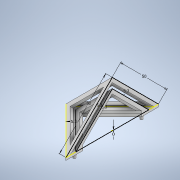
# Autodesk Inventor part: coltar5mmV3
Saved by Autodesk Inventor 2020 (Build 240168000, 168)
## iProperties
Created: 2022-02-13
Part Number: coltar5mmV3
Material: Generic
Document SubType Name: Modeling
Designer: Vlasciar
Density: 1 g/cm^3
Appearance: Default
Author: Vlasciar
Autodesk Inventor part; units mm, degrees
ref_plane "YZ Plane" through (0, 0, 0) normal (1, 0, 0) x (0, 1, 0)
ref_plane "XZ Plane" through (0, 0, 0) normal (0, 1, 0) x (-1, 0, 0)
ref_plane "XY Plane" through (0, 0, 0) normal (0, 0, 1) x (1, 0, 0)
sketch "Sketch2" plane through (0, 0, 0) normal (0, 1, 0) x (-1, 0, 0)
  line L0 (0, 35.355) -> (35.3557, 0)
  line L1 (35.3557, 0) -> (0, -35.355)
  line L2 (0, -35.355) -> (0, 35.355)
  point P0 (0, 0)
  point P1 (0, 0)
  dimension "d1" = 50
  dimension "d41" = 70.71
  constraints: 6 end point, 1 coincident, 1 equal length, 1 horizontal alignment, 1 midpoint
  measures "d1" distance of L0.start L0.end
  measures "d41" distance of L1.end L0.start
extrude "Extrusion1" add sketch "Sketch2" against normal blind 2
sketch "Sketch3" plane through (0, 0, 0) normal (0, 1, 0) x (1, 0, 0)
  line L0 (-35.3557, 0) -> (0, -35.355) projected
  line L1 (0, -35.355) -> (0, 35.355) projected
  line L2 (0, 35.355) -> (-35.3557, 0) projected
  point P0 (0, 0)
sketch "Sketch12" plane through (0, 0, 35.355) normal (1, 0, 0) x (0, 0, -1)
  line L0 (0, 0) -> (70.71, 0) projected
  line L1 (0, 0) -> (35.355, 35.3557)
  line L2 (35.355, 35.3557) -> (70.71, 0)
  line L3 (7.4953, 0) -> (63.2147, 0)
  line L4 (63.2147, 0) -> (35.355, 27.8603)
  line L5 (35.355, 27.8603) -> (7.4953, 0)
  point P0 (35.355, 0)
  dimension "d42" = 50
  dimension "d43" = 50
  dimension "d46" = 0
  dimension "d47" = 5.3
  dimension "d48" = 5.3
  constraints: 10 end point, 2 parallel, 1 horizontal
  measures "d42" distance of L1.end L0.end
  measures "d43" distance of L0.start L1.end
  measures "d46" distance between parallel lines of L0 L3
  measures "d47" distance between parallel lines of L2 L4
  measures "d48" distance between parallel lines of L1 L5
ref_plane "Work Plane5" through (-35.3557, 0, 0) normal (-0.5773466, 0.5773466, 0.5773577) x (0.7071136, 0, 0.7071)
ref_plane "Work Plane6" through (0, 0, -35.355) normal (0.5773466, -0.5773466, 0.5773577) x (-0.7071136, 0, 0.7071)
extrude "Extrusion10" add sketch "Sketch12" along normal up to surface surface through (-35.3557, 0, 0) normal (-0.5773466, 0.5773466, 0.5773577)
split "Split3" plane through (0, 0, -35.355) removes the side toward (-0.5773466, 0.5773466, -0.5773577)
shell "Shell3" thickness 2 removed faces 1 at (0, 11.7852, 0)
sketch "Sketch13" plane through (0, 0, 31.8909) normal (0, 1, 0) x (1, 0, 0)
  line L0 (-31.8916, 31.8909) -> (0, 0) projected
  line L1 (0, 63.7819) -> (0, 0) projected
  line L2 (0, 63.7819) -> (-31.8916, 31.8909) projected
  line L3 (0, 67.2459) -> (0, -3.4641) projected
  line L4 (0, 4.0312) -> (-27.8603, 31.8909)
  line L5 (-27.8603, 31.8909) -> (0, 59.7507)
  line L6 (0, -3.4641) -> (-35.3557, 31.8909) projected
  line L7 (-35.3557, 31.8909) -> (0, 67.2459) projected
  point P0 (0, 31.8909)
  dimension "d52" = 5.3
  dimension "d53" = 5.3
  constraints: 4 end point, 2 parallel, 2 point on line
  measures "d52" distance between parallel lines of L4 L6
  measures "d53" distance between parallel lines of L7 L5
ref_plane "Work Plane7" through (0, 27.8603, 0) normal (0.5773466, -0.5773466, -0.5773577) x (0, -0.7071136, 0.7071)
ref_plane "Work Plane8" through (0, 0, -27.8597) normal (-0.5773466, 0.5773466, -0.5773577) x (0, 0.7071136, 0.7071)
extrude "Extrusion11" add sketch "Sketch12" along normal up to surface separate body contours L5 L4 L0 surface through (0, 27.8603, 0) normal (0.5773466, -0.5773466, -0.5773577)
split "Split4" plane through (0, 0, -27.8597) removes the side toward (-0.5773466, 0.5773466, -0.5773577) bodies 2
shell "Shell4" thickness 2 removed faces 1 at (0, 9.2868, 0) bodies 2
sketch "Sketch14" plane through (0, 0, 35.355) normal (-0.5773466, 0.5773466, 0.5773577) x (0.8164992, 0.4082418, 0.4082496)
  line L0 (0, 50) -> (-43.3015, 24.9995) projected
  line L1 (-43.3015, 24.9995) -> (0, 0) projected
  line L2 (0, 50) -> (0, 0) projected
  line L3 (-35.3015, 24.9996) -> (-4, 43.0718)
  line L4 (-4, 43.0718) -> (-4, 6.9281)
  line L5 (-4, 6.9281) -> (-35.3015, 24.9996)
  point P0 (-14.4337, 24.9995)
  dimension "d57" = 4
  dimension "d58" = 4
  dimension "d59" = 4
  constraints: 6 end point, 3 parallel
  measures "d57" distance between parallel lines of L0 L3
  measures "d58" distance between parallel lines of L2 L4
  measures "d59" distance between parallel lines of L1 L5
extrude "Extrusion12" cut sketch "Sketch14" against normal blind 2 contours L3 L4 L5 bodies 1
sketch "Sketch15" plane through (-35.3557, 0, 0) normal (-0.5773466, 0.5773466, -0.5773577) x (-0.4082535, 0.4082535, 0.8164914)
  line L0 (-43.3011, 25.0002) -> (0, 0) projected
  line L1 (0, 50.0005) -> (0, 0) projected
  line L2 (-43.3011, 25.0002) -> (0, 50.0005) projected
  line L3 (-4, 43.0722) -> (-4, 6.9282)
  line L4 (-4, 6.9282) -> (-35.3012, 25.0002)
  line L5 (-35.3012, 25.0002) -> (-4, 43.0722)
  point P0 (-14.4341, 25.0002)
  dimension "d62" = 4
  dimension "d63" = 4
  dimension "d64" = 4
  constraints: 6 end point, 3 parallel
  measures "d62" distance between parallel lines of L2 L5
  measures "d63" distance between parallel lines of L1 L3
  measures "d64" distance between parallel lines of L0 L4
extrude "Extrusion13" cut sketch "Sketch15" against normal blind 2 contours L3 L4 L5 bodies 1
sketch "Sketch16" plane through (-27.8603, 0, 0) normal (-0.5773466, 0.5773466, -0.5773577) x (-0.4082535, 0.4082535, 0.8164914)
  line L0 (0, 0) -> (-34.1213, 19.7002) projected
  line L1 (0, 39.4004) -> (0, 0) projected
  line L2 (-34.1213, 19.7002) -> (0, 39.4004) projected
  line L3 (-4, 32.4721) -> (-4, 6.9282)
  line L4 (-4, 6.9282) -> (-26.1214, 19.7002)
  line L5 (-26.1214, 19.7002) -> (-4, 32.4721)
  point P0 (-11.3741, 19.7002)
  dimension "d67" = 4
  dimension "d68" = 4
  dimension "d69" = 4
  constraints: 6 end point, 3 parallel
  measures "d67" distance between parallel lines of L0 L4
  measures "d68" distance between parallel lines of L2 L5
  measures "d69" distance between parallel lines of L1 L3
extrude "Extrusion14" cut sketch "Sketch16" against normal blind 2 contours L3 L4 L5 bodies 2
sketch "Sketch17" plane through (-27.8603, 0, 0) normal (-0.5773466, 0.5773466, 0.5773577) x (0.4082535, -0.4082535, 0.8164914)
  line L0 (0, 39.4004) -> (0, 0) projected
  line L1 (0, 0) -> (34.1213, 19.7002) projected
  line L2 (34.1213, 19.7002) -> (0, 39.4004) projected
  line L3 (4, 6.9282) -> (4, 32.4721)
  line L4 (4, 32.4721) -> (26.1214, 19.7002)
  line L5 (26.1214, 19.7002) -> (4, 6.9282)
  point P0 (11.3741, 19.7002)
  dimension "d72" = 4
  dimension "d73" = 4
  dimension "d74" = 4
  constraints: 6 end point, 3 parallel
  measures "d72" distance between parallel lines of L0 L3
  measures "d73" distance between parallel lines of L2 L4
  measures "d74" distance between parallel lines of L1 L5
extrude "Extrusion15" cut sketch "Sketch17" against normal blind 2 contours L3 L4 L5 bodies 2
sketch "Sketch18" plane through (0, 2, 22.3957) normal (0, 1, 0) x (1, 0, 0)
  line L0 (-22.3962, 22.3957) -> (0, 44.7914) projected
  line L1 (-22.3962, 22.3957) -> (0, 0) projected
  line L2 (0, 44.7914) -> (0, 0) projected
  point P0 (0, 22.3957)
extrude "Extrusion16" cut sketch "Sketch18" against normal blind 4 bodies 2 1
sketch "Sketch19" plane through (0, -2, 0) normal (0, -1, 0) x (1, 0, 0)
  circle A0 centre (-3.6588, 25.1048) radius 1
  line L0 (-2.1113, -27.6684) -> (-27.669, -2.1113) projected
  circle A1 centre (-3.6588, -26.121) radius 1
  line L1 (0, 0) -> (-35.3557, 0) projected
  circle A2 centre (-28.5731, 0) radius 1
  dimension "d79" = 2
  dimension "d80" = 2
  dimension "d81" = 2
  constraints: 3 centre point, 2 point on line
  measures "d79" diameter of A0
  measures "d80" diameter of A1
  measures "d81" diameter of A2
extrude "Extrusion17" add sketch "Sketch19" along normal blind 5 bodies 1
draft "FaceDraft2" angle 10 pull direction (0, -1, 0) faces at (-27.586, -5.3333, -0.1604) (-4.4582, -5.3333, -26.7217) (-2.7103, -5.3333, 24.7881) fixed edges at (-29.5731, -7, 0) (-4.6588, -7, -26.121) (-4.6588, -7, 25.1048)
body "Solid1"
body "Solid3"
